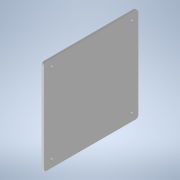
# Autodesk Inventor part: Plate
Saved by Autodesk Inventor 2022 (Build 260153000, 153)
## iProperties
Created: 2022-03-14
Part Number: Plate
Material: Generic
Document SubType Name: Modeling
Designer: ultra
Density: 1 g/cm^3
Appearance: Default
Author: ultra
Autodesk Inventor part; units mm, degrees
ref_plane "YZ Plane" through (0, 0, 0) normal (1, 0, 0) x (0, 1, 0)
ref_plane "XZ Plane" through (0, 0, 0) normal (0, 1, 0) x (-1, 0, 0)
ref_plane "XY Plane" through (0, 0, 0) normal (0, 0, 1) x (1, 0, 0)
sketch "Sketch1" plane through (0, 0, 0) normal (1, 0, 0) x (0, 1, 0)
  circle A0 centre (-53.8421, 54.0138) radius 2.032
  circle A1 centre (53.921, -53.7492) radius 2.032
  circle A2 centre (0.0394, -76.0677) radius 2.032
  circle A3 centre (53.921, 54.0138) radius 2.032
  circle A4 centre (-76.1606, 0.1323) radius 2.032
  circle A5 centre (76.2394, 0.1323) radius 2.032
  circle A6 centre (-53.8421, -53.7492) radius 2.032
  circle A7 centre (0.0394, 76.3323) radius 2.032
  line L0 (-63.5, 63.5) -> (63.5, 63.5)
  line L1 (63.5, 63.5) -> (63.5, -63.5)
  line L2 (63.5, -63.5) -> (-63.5, -63.5)
  line L3 (-63.5, -63.5) -> (-63.5, 63.5)
  line L4 (-63.5, 63.5) -> (63.5, -63.5) construction
  line L5 (63.5, 63.5) -> (-63.5, -63.5) construction
  point P0 (0, 0)
  dimension "d0" = 127
  dimension "d1" = 127
  constraints: 12 end point, 8 centre point, 2 midpoint, 2 parallel, 1 horizontal, 1 perpendicular
  measures "d0" distance of L1.end L2.end
  measures "d1" distance of L0.end L1.end
extrude "Extrusion1" add sketch "Sketch1" along normal blind 3.175 contours L0 L1 L2 L3
fillet "Fillet1" radius 3.175 4 edges at (1.5875, -63.5, 63.5) (1.5875, -63.5, -63.5) (1.5875, 63.5, -63.5) (1.5875, 63.5, 63.5)
body "Solid1"
